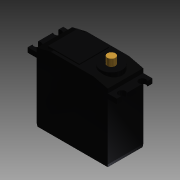
# Autodesk Inventor part: ServoModel
Saved by Autodesk Inventor 2014 (Build 180170000, 170)
## iProperties
Created: 2014-02-24
Part Number: ServoModel
Material: Generic
Document SubType Name: Modeling
Designer: Jonathan
Density: 1 g/cm^3
Appearance: Default
Author: Jonathan
Autodesk Inventor part; units mm, degrees
ref_plane "YZ Plane" through (0, 0, 0) normal (1, 0, 0) x (0, 1, 0)
ref_plane "XZ Plane" through (0, 0, 0) normal (0, 1, 0) x (-1, 0, 0)
ref_plane "XY Plane" through (0, 0, 0) normal (0, 0, 1) x (1, 0, 0)
sketch "Sketch1" plane through (0, 0, 0) normal (0, 1, 0) x (-1, 0, 0)
  line L0 (0, -23.3131) -> (0, 24.6505)
  line L1 (49.2542, 0) -> (-47.6933, 0)
  arc A0 (37.265, -6.345) -> (37.265, -10.765) centre (35.3109, -8.555) ccw
  line L2 (37.265, -14.815) -> (37.265, -10.765)
  arc A1 (37.265, 10.765) -> (37.265, 6.345) centre (35.3109, 8.555) ccw
  line L3 (37.265, 14.815) -> (37.265, 10.765)
  line L4 (37.265, -6.345) -> (37.265, 6.345)
  line L5 (37.265, -14.815) -> (29.695, -14.815)
  line L6 (37.265, 14.815) -> (29.695, 14.815)
  arc A2 (-37.265, -10.765) -> (-37.265, -6.345) centre (-35.3109, -8.555) ccw
  line L7 (-37.265, -14.815) -> (-37.265, -10.765)
  line L8 (-37.265, 14.815) -> (-37.265, 10.765)
  arc A3 (-37.265, 6.345) -> (-37.265, 10.765) centre (-35.3109, 8.555) ccw
  line L9 (-37.265, -6.345) -> (-37.265, 6.345)
  line L10 (-37.265, -14.815) -> (-29.695, -14.815)
  line L11 (-37.265, 14.815) -> (-29.695, 14.815)
  line L12 (29.695, -14.815) -> (-29.695, -14.815)
  line L13 (-29.695, 14.815) -> (29.695, 14.815)
  line L14 (29.695, -14.815) -> (29.695, 14.815)
  line L15 (-29.695, -14.815) -> (-29.695, 14.815)
  point P0 (0, 0)
  dimension "d3" = 4.42
  dimension "d6" = 2.95
  dimension "d7" = 7.57
  dimension "d8" = 3.31
  dimension "d9" = 59.39
  dimension "d10" = 29.63
  constraints: 32 end point, 13 symmetric about line, 8 point on circle, 4 centre point, 4 collinear, 3 perpendicular, 2 point on line, 1 vertical, 3 other
  measures "d3" distance of L4.start L2.end
  measures "d6" radius of A0
  measures "d7" distance of L3.start L6.end
  measures "d8" distance edge to line of A0 L5
  measures "d9" distance between parallel lines of L15 L14
  measures "d10" distance between parallel lines of L13 L12
extrude "Extrusion1" add sketch "Sketch1" along normal blind 3.95
sketch "Sketch2" plane through (0, 3.95, 0) normal (0, 1, 0) x (1, 0, 0)
  line L0 (37.265, 14.815) -> (-37.265, 14.815) projected
  line L1 (-37.265, -14.815) -> (37.265, -14.815) projected
  line L2 (-29.695, 14.815) -> (29.695, 14.815)
  line L3 (29.695, 14.815) -> (29.695, -14.815)
  line L4 (29.695, -14.815) -> (-29.695, -14.815)
  line L5 (-29.695, -14.815) -> (-29.695, 14.815)
  point P0 (0, 0)
  dimension "d13" = 59.39
  dimension "d14" = 29.695
  constraints: 8 end point, 2 parallel, 2 point on line, 1 horizontal, 1 perpendicular
  measures "d13" distance between parallel lines of L3 L5
  measures "d14" distance from line of point (0, 0) L3
extrude "Extrusion2" add sketch "Sketch2" along normal blind 3.5
sketch "Sketch3" plane through (0, 0, 0) normal (0, -1, 0) x (1, 0, 0)
  line L0 (37.265, -14.815) -> (-37.265, -14.815) projected
  line L1 (-37.265, 14.815) -> (37.265, 14.815) projected
  line L2 (-29.695, 14.815) -> (29.695, 14.815)
  line L3 (29.695, 14.815) -> (29.695, -14.815)
  line L4 (29.695, -14.815) -> (-29.695, -14.815)
  line L5 (-29.695, -14.815) -> (-29.695, 14.815)
  point P0 (0, 0)
  dimension "d17" = 59.39
  dimension "d18" = 29.695
  constraints: 8 end point, 2 parallel, 2 point on line, 1 horizontal, 1 perpendicular
  measures "d17" distance between parallel lines of L3 L5
  measures "d18" distance from line of point (0, 0) L5
extrude "Extrusion3" add sketch "Sketch3" along normal blind 49.69
sketch "Sketch4" plane through (37.265, 0, 14.815) normal (0, 0, 1) x (1, 0, 0)
  line L0 (-7.57, -49.69) -> (-66.96, -49.69) projected
  line L1 (-66.96, 7.45) -> (-7.57, 7.45) projected
  line L2 (-74.53, 0) -> (-74.53, 3.95) projected
  line L3 (-66.96, 7.45) -> (-55.11, 10.31)
  line L4 (-55.11, 10.31) -> (-19.42, 10.31)
  line L5 (-19.42, 10.31) -> (-7.57, 7.45)
  line L6 (14.6439, 12.17) -> (-93.8376, 12.17) construction
  line L7 (-75.1527, 11.11) -> (-5.1295, 11.11) construction
  point P0 (-37.265, 0)
  dimension "d21" = 11.85
  dimension "d22" = 11.85
  dimension "d31" = 1.06
  dimension "d32" = 0.8
  dimension "d44" = 60.8
  constraints: 10 end point, 2 parallel, 1 perpendicular
  measures "d21" horizontal distance of L1.end L4.end
  measures "d22" horizontal distance of L1.start L3.end
  measures "d31" distance between parallel lines of L6 L7
  measures "d32" distance between parallel lines of L4 L7
  measures "d44" distance between parallel lines of L7 L0
sketch "Sketch5" plane through (0, 7.45, 0) normal (0, 1, 0) x (1, 0, 0)
  line L0 (29.695, -14.815) -> (29.695, 14.815) projected
  line L1 (29.695, 14.815) -> (-29.695, 14.815) projected
  circle A0 centre (17.845, 0) radius 9
  point P0 (0, 0)
  dimension "d23" = 11.85
  dimension "d24" = 18
  dimension "d29" = 14.815
  constraints: 1 centre point
  measures "d23" distance from line of L0 A0.centre
  measures "d24" diameter of A0
  measures "d29" distance from line of A0.centre L1
extrude "Extrusion4" add sketch "Sketch5" along normal blind 4.72
sketch "Sketch6" plane through (0, 7.45, 0) normal (0, 1, 0) x (1, 0, 0)
  line L0 (-29.695, 14.815) -> (-29.695, -14.815) projected
  line L1 (-22.695, 12.5) -> (3.505, 12.5)
  line L2 (3.505, 12.5) -> (3.505, -12.5)
  line L3 (3.505, -12.5) -> (-22.695, -12.5)
  line L4 (-22.695, -12.5) -> (-22.695, 12.5)
  line L5 (-37.265, 6.345) -> (-37.265, -6.345) projected
  point P0 (0, 0)
  dimension "d35" = 25
  dimension "d36" = 12.5
  dimension "d38" = 26.2
  dimension "d39" = 7
  constraints: 8 end point, 2 parallel, 1 horizontal, 1 perpendicular
  measures "d35" distance of L3.end L1.start
  measures "d36" distance from line of L1 point (0, 0)
  measures "d38" distance of L1.start L1.end
  measures "d39" distance between parallel lines of L4 L0
extrude "Extrusion5" add sketch "Sketch6" along normal blind 3.66
extrude "Extrusion6" add sketch "Sketch4" against normal up to surface (29.63 mm away)
sketch "Sketch7" plane through (17.845, 12.17, 0) normal (0, 1, 0) x (1, 0, 0)
  circle A0 centre (0, 0) radius 9 projected
  circle A1 centre (0, 0) radius 3.365
  point P0 (-17.845, 0)
  dimension "d45" = 6.73
  constraints: 1 centre point, 1 coincident
  measures "d45" diameter of A1
extrude "Extrusion7" add sketch "Sketch7" along normal blind 5.95 contours A1
chamfer "Chamfer1" distance 0.25 distance2 2.2 1 edges at (0, -49.69, -14.815) measured on face at (-9.8983, -49.69, 4.9383)
chamfer "Chamfer2" distance 0.25 distance2 2.2 1 edges at (0, -49.69, 14.815) measured on face at (9.8983, -49.69, -4.7717)
chamfer "Chamfer3" distance 0.25 distance2 2.2 1 edges at (29.695, -49.69, 0) measured on face at (-9.8983, -49.69, 4.855)
chamfer "Chamfer4" distance 0.25 distance2 2.2 1 edges at (-29.695, -49.69, 0) measured on face at (-9.9817, -49.69, 4.855)
equation "\"d13\" = d9"
equation "\"d14\" = 0.5 * d9"
equation "\"d17\" = d9"
equation "\"d18\" = 0.5 * d9"
equation "\"d22\" = d21"
equation "\"d29\" = 0.5 * d10"
equation "\"d36\" = 0.5 * d35"
body "Solid1"
